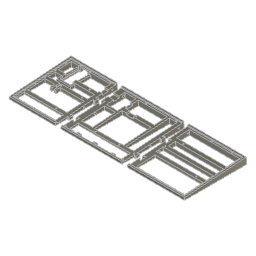
pavilion-x360-keyboard (Autodesk Fusion 360 design; units mm, degrees)
Autodesk Fusion 360 part; units mm, degrees
note: some values were not read from the file. Set by a fixed rule: which face or edge a step refers to.
(part 1 of 2)
ref_plane "WorkPlane3" through (12.125, 0, 0) normal (0, -0.069756, 0.997564) x (1, 0, 0)
sketch "Top" plane through (0, 0, 0) normal (0, -0.069756, 0.997564) x (1, 0, 0)
  line L0 (83, 3) -> (83, 0)
  line L1 (83, 0) -> (0, 0)
  line L2 (0, 0) -> (0, 111.5)
  line L3 (0, 111.5) -> (83, 111.5)
  line L4 (83, 111.5) -> (83, 108.5)
  line L5 (3, 99) -> (4, 99)
  arc A0 (3.9974, 97) -> (4, 99) centre (4, 98) ccw
  line L6 (3.9974, 97) -> (3, 97)
  line L7 (3, 80.5) -> (4, 80.5)
  line L8 (3, 62) -> (4, 62)
  arc A1 (4, 60) -> (4, 62) centre (4, 61) ccw
  line L9 (4, 60) -> (3, 60)
  line L10 (3, 43.5) -> (4, 43.5)
  line L11 (20, 108.5) -> (20, 107.5)
  line L12 (22, 107.5) -> (22, 108.5)
  line L13 (38, 108.5) -> (38, 107.5)
  line L14 (40, 107.5) -> (40, 108.5)
  line L15 (74.5, 108.5) -> (74.5, 107.5)
  line L16 (6.25, 3) -> (6.25, 4)
  line L17 (8.25, 4) -> (8.25, 3)
  line L18 (40.5, 3) -> (40.5, 4)
  line L19 (42.5, 4) -> (42.5, 3)
  line L20 (59.25, 3) -> (59.25, 4)
  line L21 (61.25, 4) -> (61.25, 3)
  line L22 (83, 108.5) -> (76.5, 108.5)
  line L23 (74.5, 108.5) -> (40, 108.5)
  line L24 (38, 108.5) -> (22, 108.5)
  line L25 (20, 108.5) -> (3, 108.5)
  line L26 (3, 108.5) -> (3, 99)
  line L27 (3, 97) -> (3, 80.5)
  line L28 (3, 78.5) -> (3, 62)
  line L29 (3, 60) -> (3, 43.5)
  line L30 (3, 41.5) -> (3, 25)
  line L31 (3, 23) -> (3, 3)
  line L32 (3, 3) -> (6.25, 3)
  line L33 (8.25, 3) -> (21.75, 3)
  line L34 (23.75, 3) -> (40.5, 3)
  line L35 (42.5, 3) -> (59.25, 3)
  line L36 (61.25, 3) -> (83, 3)
  line L37 (93, 3) -> (93, 0)
  line L38 (93, 0) -> (203.25, 0)
  line L39 (203.25, 0) -> (203.25, 3)
  line L40 (97.25, 3) -> (97.25, 4)
  arc A2 (99.25, 4) -> (97.25, 4) centre (98.25, 4) ccw
  line L41 (99.25, 4) -> (99.25, 3)
  line L42 (118.25, 3) -> (118.25, 4)
  arc A3 (120.25, 4) -> (118.25, 4) centre (119.25, 4) ccw
  line L43 (120.25, 4) -> (120.25, 3)
  line L44 (147.75, 3) -> (147.75, 4)
  arc A4 (149.75, 4) -> (147.75, 4) centre (148.75, 4) ccw
  line L45 (149.75, 4) -> (149.75, 3)
  line L46 (181.25, 3) -> (181.25, 4)
  arc A5 (183.25, 4) -> (181.25, 4) centre (182.25, 4) ccw
  line L47 (183.25, 4) -> (183.25, 3)
  line L48 (116.25, 3) -> (116.25, 2.5)
  line L49 (116.25, 2.5) -> (110.25, 2.5)
  line L50 (110.25, 2.5) -> (110.25, 3)
  line L51 (122.25, 3) -> (122.25, 2.5)
  line L52 (122.25, 2.5) -> (145.75, 2.5)
  line L53 (145.75, 2.5) -> (145.75, 3)
  line L54 (179.25, 3) -> (179.25, 2.5)
  line L55 (179.25, 2.5) -> (151.75, 2.5)
  line L56 (151.75, 2.5) -> (151.75, 3)
  line L57 (197.25, 3) -> (197.25, 2.5)
  line L58 (197.25, 2.5) -> (185.25, 2.5)
  line L59 (185.25, 2.5) -> (185.25, 3)
  line L60 (97.25, 3) -> (93, 3)
  line L61 (118.25, 3) -> (116.25, 3)
  line L62 (110.25, 3) -> (99.25, 3)
  line L63 (147.75, 3) -> (145.75, 3)
  line L64 (122.25, 3) -> (120.25, 3)
  line L65 (151.75, 3) -> (149.75, 3)
  line L66 (181.25, 3) -> (179.25, 3)
  line L67 (185.25, 3) -> (183.25, 3)
  line L68 (203.25, 3) -> (201.25, 3)
  line L69 (199.25, 3) -> (197.25, 3)
  line L70 (93, 111.5) -> (203.25, 111.5)
  line L71 (203.25, 111.5) -> (203.25, 108.5)
  line L72 (93, 108.5) -> (93, 111.5)
  line L73 (138.75, 108.5) -> (138.75, 107.5)
  line L74 (140.75, 107.5) -> (140.75, 108.5)
  line L75 (193.25, 108.5) -> (193.25, 107.5)
  line L76 (195.25, 107.5) -> (195.25, 108.5)
  line L77 (138.75, 108.5) -> (93, 108.5)
  line L78 (203.25, 108.5) -> (195.25, 108.5)
  line L79 (193.25, 108.5) -> (140.75, 108.5)
  line L80 (213.25, 108.5) -> (213.25, 111.5)
  line L81 (213.25, 111.5) -> (316.25, 111.5)
  line L82 (316.25, 111.5) -> (316.25, 0)
  line L83 (316.25, 0) -> (213.25, 0)
  line L84 (213.25, 0) -> (213.25, 3)
  line L85 (313.25, 99) -> (312.25, 99)
  line L86 (313.25, 62) -> (312.25, 62)
  line L87 (313.25, 43.5) -> (312.25, 43.5)
  arc A6 (312.25, 43.5) -> (312.2531, 41.5) centre (312.25, 42.5) ccw
  line L88 (312.2531, 41.5) -> (313.25, 41.5)
  line L89 (313.25, 25) -> (312.25, 25)
  arc A7 (312.25, 25) -> (312.25, 23) centre (312.25, 24) ccw
  line L90 (312.25, 23) -> (313.25, 23)
  line L91 (313.25, 99) -> (313.25, 108.5)
  line L92 (313.25, 80.5) -> (313.25, 97)
  line L93 (313.25, 62) -> (313.25, 78.5)
  line L94 (313.25, 3) -> (313.25, 23)
  line L95 (313.25, 25) -> (313.25, 41.5)
  line L96 (313.25, 43.5) -> (313.25, 60)
  line L97 (308, 3) -> (308, 4)
  arc A8 (310, 4) -> (308, 4) centre (309, 4) ccw
  line L98 (310, 4) -> (310, 3)
  line L99 (293.5, 3) -> (293.5, 4)
  arc A9 (295.5, 4) -> (293.5, 4) centre (294.5, 4) ccw
  line L100 (295.5, 4) -> (295.5, 3)
  line L101 (256, 3) -> (256, 4)
  arc A10 (258, 4) -> (256, 4) centre (257, 4) ccw
  line L102 (258, 4) -> (258, 3)
  line L103 (293.5, 108.5) -> (293.5, 107.4999)
  line L104 (295.5, 107.5) -> (295.5, 108.5)
  line L105 (257, 108.5) -> (257, 107.5)
  line L106 (259, 107.5) -> (259, 108.5)
  line L107 (213.25, 3) -> (256, 3)
  line L108 (258, 3) -> (293.5, 3)
  line L109 (295.5, 3) -> (308, 3)
  line L110 (310, 3) -> (313.25, 3)
  line L111 (257, 108.5) -> (213.25, 108.5)
  line L112 (313.25, 108.5) -> (295.5, 108.5)
  line L113 (293.5, 108.5) -> (259, 108.5)
  line L114 (4, 98) -> (312.25, 98) construction
  line L115 (313.25, 111.5) -> (313.25, 0) construction
  arc A11 (312.25, 99) -> (312.2477, 97) centre (312.25, 98) ccw
  line L116 (312.2477, 97) -> (313.25, 97)
  line L117 (4, 79.5) -> (312.25, 79.5) construction
  line L118 (313.25, 80.5) -> (312.25, 80.5)
  line L119 (313.25, 78.5) -> (312.2478, 78.5)
  arc A12 (312.25, 80.5) -> (312.2478, 78.5) centre (312.25, 79.5) ccw
  line L120 (4, 42.5) -> (312.25, 42.5) construction
  line L121 (4, 24) -> (312.25, 24) construction
  line L122 (0, 108.5) -> (316.25, 108.5) construction
  line L123 (0, 3) -> (316.25, 3) construction
  line L124 (3, 0) -> (3, 111.5) construction
  line L125 (93, 2.5) -> (203.25, 2.5) construction
  arc A13 (312.25, 62) -> (312.2508, 60) centre (312.25, 61) ccw
  line L126 (312.2508, 60) -> (313.25, 60)
  line L127 (4, 61) -> (312.25, 61) construction
  arc A14 (20, 107.5) -> (22, 107.5) centre (21, 107.5) ccw
  arc A15 (38, 107.5) -> (40, 107.5) centre (39, 107.5) ccw
  arc A16 (61.25, 4) -> (59.25, 4) centre (60.25, 4) ccw
  arc A17 (293.5, 107.4999) -> (295.5, 107.5) centre (294.5, 107.4999) ccw
  arc A18 (257, 107.5) -> (259, 107.5) centre (258, 107.5) ccw
  line L128 (3, 78.5) -> (4.0035, 78.5)
  arc A19 (4.0035, 78.5) -> (4, 80.5) centre (4, 79.5) ccw
  line L129 (3, 25) -> (4, 25)
  line L130 (3, 23) -> (4.0015, 23)
  line L131 (3, 41.5) -> (3.9975, 41.5)
  arc A20 (3.9975, 41.5) -> (4, 43.5) centre (4, 42.5) ccw
  arc A21 (4.0015, 23) -> (4, 25) centre (4, 24) ccw
  arc A22 (193.25, 107.5) -> (195.25, 107.5) centre (194.25, 107.5) ccw
  arc A23 (138.75, 107.5) -> (140.75, 107.5) centre (139.75, 107.5) ccw
  line L132 (199.25, 3) -> (199.25, 4)
  line L133 (201.25, 3) -> (201.25, 4)
  arc A24 (201.25, 4) -> (199.25, 4) centre (200.25, 4) ccw
  line L134 (76.5, 108.5) -> (76.5, 107.5)
  arc A25 (74.5, 107.5) -> (76.5, 107.5) centre (75.5, 107.5) ccw
  arc A26 (8.25, 4) -> (6.25, 4) centre (7.25, 4) ccw
  arc A27 (42.5, 4) -> (40.5, 4) centre (41.5, 4) ccw
  line L135 (21.75, 3) -> (21.75, 4)
  arc A28 (23.75, 4) -> (21.75, 4) centre (22.75, 4) ccw
  line L136 (23.75, 4) -> (23.75, 3)
  dimension "d87" = 105.5
  dimension "d91" = 3
  dimension "d93" = 1
  dimension "d227" = 1
  dimension "d235" = 1
  dimension "d238" = 1
  dimension "d259" = 1
  dimension "d261" = 1
  dimension "d322" = 1
  dimension "d323" = 1
  dimension "d324" = 1
  dimension "d325" = 4.25
  dimension "d326" = 14.5
  dimension "d327" = 37.5
  dimension "d343" = 10
  dimension "d383" = 2
  dimension "d390" = 2
  dimension "d391" = 2
  dimension "d393" = 100
  dimension "d395" = 3
  dimension "d396" = 1
  dimension "d399" = 1
  dimension "d402" = 1
  dimension "d403" = 2
  dimension "d412" = 3
  dimension "d415" = 3
  dimension "d417" = 0.5
  dimension "d419" = 1
  dimension "d444" = 34.5
  dimension "d445" = 17.75
  dimension "d446" = 9.5
  dimension "d447" = 16.5
  dimension "d448" = 16.5
  dimension "d460" = 1
  dimension "d461" = 1
  dimension "d543" = 1
  dimension "d544" = 17
  dimension "d545" = 2
  dimension "d548" = 16
  dimension "d549" = 2
  dimension "d550" = 34.5
  dimension "d554" = 1
  dimension "d555" = 1
  dimension "d568" = 1
  dimension "d569" = 1
  dimension "d570" = 2
  dimension "d571" = 1
  dimension "d572" = 1
  dimension "d573" = 2
  dimension "d574" = 1
  dimension "d575" = 1
  dimension "d576" = 2
  dimension "d577" = 2
  dimension "d578" = 1
  dimension "d579" = 2
  dimension "d580" = 1
  dimension "d581" = 16.5
  dimension "d582" = 2
  dimension "d583" = 1
  dimension "d585" = 9.5
  dimension "d587" = 1
  dimension "d588" = 2
  dimension "d590" = 1
  dimension "d592" = 16.5
  dimension "d594" = 2
  dimension "d595" = 1
  dimension "d596" = 16.5
  dimension "d598" = 1
  dimension "d600" = 2
  dimension "d601" = 1
  dimension "d602" = 1
  dimension "d603" = 16.5
  dimension "d611" = 1
  dimension "d615" = 2
  dimension "d617" = 1
  dimension "d618" = 2
  dimension "d619" = 16.5
  dimension "d620" = 1
  dimension "d621" = 20
  dimension "d626" = 2
  dimension "d627" = 4.25
  dimension "d628" = 11
  dimension "d629" = 2
  dimension "d630" = 2
  dimension "d631" = 23.5
  dimension "d632" = 2
  dimension "d633" = 2
  dimension "d634" = 27.5
  dimension "d635" = 2
  dimension "d636" = 2
  dimension "d637" = 2
  dimension "d638" = 12
  dimension "d641" = 2
  dimension "d643" = 6
  dimension "d644" = 2
  dimension "d646" = 2
  dimension "d649" = 10
  dimension "d650" = 1
  dimension "d651" = 2
  dimension "d653" = 2
  dimension "d654" = 2
  dimension "d655" = 2
  dimension "d760" = 22.75
  dimension "d762" = 18.75
  dimension "d766" = 1
  dimension "d767" = 4.25
  dimension "d768" = 1
  dimension "d769" = 1
  dimension "d771" = 1
  dimension "d772" = 15.5
  dimension "d773" = 1
  dimension "d774" = 18.75
  dimension "d775" = 1
  dimension "d776" = 9
  dimension "d779" = 2
  dimension "d781" = 46.75
  constraint perpendicular L0 L1
  constraint tangent L5 A0
  constraint coincident L6.end L26
  constraint coincident L7.start L26
  constraint coincident L8.start L26
  constraint tangent L8 A1
  constraint coincident L9.end L26
  constraint coincident L10.start L26
  constraint coincident L1.end L2.start
  constraint coincident L30.start L26
  constraint coincident L30.end L26
  constraint coincident L31.start L26
  constraint coincident L11.start L22
  constraint coincident L12.end L22
  constraint coincident L13.start L22
  constraint coincident L14.end L22
  constraint coincident L15.start L22
  constraint coincident L17.end L32
  constraint coincident L28.start L26
  constraint coincident L33.end L32
  constraint coincident L34.start L32
  constraint coincident L18.start L32
  constraint coincident L19.end L32
  constraint coincident L20.start L32
  constraint coincident L21.end L32
  constraint coincident L40.start L68
  constraint tangent L40 A2
  constraint tangent A2 L41
  constraint coincident L42.start L68
  constraint tangent L42 A3
  constraint tangent A3 L43
  constraint coincident L44.start L68
  constraint tangent L44 A4
  constraint tangent A4 L45
  constraint coincident L46.start L68
  constraint tangent L46 A5
  constraint tangent A5 L47
  constraint coincident L69.start L68
  constraint collinear L1 L38
  constraint coincident L50.end L68
  constraint coincident L53.end L68
  constraint coincident L56.end L68
  constraint coincident L59.end L68
  constraint horizontal L78
  constraint collinear L3 L70
  constraint collinear L37 L72
  constraint collinear L39 L71
  constraint coincident L73.start L78
  constraint coincident L75.start L78
  constraint collinear L77 L78
  constraint collinear L78 L79
  constraint perpendicular L39 L107
  constraint perpendicular L71 L112
  constraint perpendicular L70 L80
  constraint perpendicular L71 L81
  constraint perpendicular L39 L83
  constraint perpendicular L84 L107
  constraint coincident L85.start L94
  constraint coincident L92.start L94
  constraint coincident L86.start L94
  constraint coincident L87.start L94
  constraint tangent L87 A6
  constraint coincident L88.end L94
  constraint coincident L89.start L94
  constraint tangent L89 A7
  constraint tangent A7 L90
  constraint collinear L3 L81
  constraint collinear L1 L83
  constraint collinear L80 L84
  constraint coincident L97.start L107
  constraint vertical L97
  constraint tangent L97 A8
  constraint coincident L98.end L107
  constraint tangent A8 L98
  constraint perpendicular L98 L107
  constraint coincident L99.start L107
  constraint perpendicular L99 L107
  constraint tangent L99 A9
  constraint coincident L100.end L107
  constraint tangent A9 L100
  constraint perpendicular L100 L107
  constraint perpendicular L101 L107
  constraint tangent L101 A10
  constraint coincident L102.end L107
  constraint tangent A10 L102
  constraint perpendicular L102 L107
  constraint coincident L103.start L112
  constraint coincident L105.start L112
  constraint collinear L108 L109
  constraint collinear L109 L110
  constraint collinear L111 L112
  constraint collinear L112 L113
  constraint coincident A0.centre L114.start
  constraint coincident L81 L115.start
  constraint coincident L83 L115.end
  constraint perpendicular L83 L115
  constraint collinear L91 L115
  constraint collinear L92 L115
  constraint collinear L93 L115
  constraint collinear L96 L115
  constraint tangent L85 A11
  constraint coincident L114 A11.centre
  constraint horizontal L117
  constraint tangent L118 A12
  constraint coincident L117 A12.centre
  constraint perpendicular L89 L95
  constraint perpendicular L90 L94
  constraint horizontal L120
  constraint coincident A6.centre L120
  constraint horizontal L114
  constraint horizontal L121
  constraint coincident A7.centre L121
  constraint coincident L3 L124.end
  constraint coincident L2 L122.start
  constraint coincident L2 L123.start
  constraint perpendicular L0 L123
  constraint collinear L32 L123
  constraint coincident L1 L124.start
  constraint perpendicular L3 L124
  constraint collinear L31 L124
  constraint collinear L30 L124
  constraint collinear L29 L124
  constraint perpendicular L2 L122
  constraint collinear L25 L122
  constraint collinear L24 L122
  constraint collinear L0 L4
  constraint collinear L77 L122
  constraint collinear L111 L122
  constraint collinear L60 L123
  constraint collinear L62 L123
  constraint collinear L36 L123
  constraint collinear L61 L123
  constraint collinear L64 L123
  constraint collinear L65 L123
  constraint collinear L66 L123
  constraint collinear L67 L123
  constraint coincident L37 L125.start
  constraint perpendicular L39 L125
  constraint coincident L39 L125.end
  constraint collinear L49 L125
  constraint collinear L52 L125
  constraint collinear L55 L125
  constraint collinear L58 L125
  constraint collinear L69 L123
  constraint collinear L107 L123
  constraint tangent L86 A13
  constraint coincident A1.centre L127
  constraint tangent L11 A14
  constraint tangent L13 A15
  constraint tangent L20 A16
  constraint tangent L103 A17
  constraint tangent L105 A18
  constraint coincident L7.start L124
  constraint tangent L7 A19
  constraint coincident L117.start A19.centre
  constraint coincident A1.centre L127.start
  constraint horizontal L127
  constraint tangent L10 A20
  constraint coincident L120.start A20.centre
  constraint tangent L129 A21
  constraint coincident L121.start A21.centre
  constraint tangent L75 A22
  constraint tangent L76 A22
  constraint tangent L73 A23
  constraint tangent L74 A23
  constraint tangent L14 A15
  constraint tangent L12 A14
  constraint tangent L21 A16
  constraint tangent L132 A24
  constraint tangent L133 A24
  constraint tangent L15 A25
  constraint tangent L134 A25
  constraint tangent L16 A26
  constraint tangent L17 A26
  constraint coincident L82 L122.end
  constraint coincident L114.end A11.centre
  constraint coincident L117.end A12.centre
  constraint coincident A13.centre L127.end
  constraint coincident A6.centre L120.end
  constraint coincident A7.centre L121.end
  constraint coincident L82 L123.end
  constraint tangent L18 A27
  constraint tangent L19 A27
  constraint perpendicular L16 L32
  constraint perpendicular L17 L33
  constraint perpendicular L33 L135
  constraint tangent L135 A28
  constraint perpendicular L18 L34
  constraint perpendicular L19 L35
  constraint perpendicular L20 L35
  constraint perpendicular L21 L36
  constraint tangent A28 L136
  constraint perpendicular L34 L136
  constraint perpendicular L75 L79
  constraint perpendicular L73 L77
  measures "d87" distance of L25.end L31.end
  measures "d91" distance of L4.end L3.end
  measures "d93" distance of L5.start L5.end
  measures "d227" distance of L42.start L42.end
  measures "d235" distance of L44.start L44.end
  measures "d238" distance of L46.start L46.end
  measures "d259" distance of L73.start L73.end
  measures "d261" distance of L75.start L75.end
  measures "d322" distance of L97.start L97.end
  measures "d323" distance of L99.start L99.end
  measures "d324" distance of L101.start L101.end
  measures "d325" distance of L94 A8.centre
  measures "d326" distance of A8.centre A9.centre
  measures "d327" distance of A9.centre A10.centre
  measures "d343" distance of L39 L84
  measures "d383" distance of L101.end A10.start
  measures "d390" distance of L99.end A9.start
  measures "d391" distance of L97.end A8.start
  measures "d393" distance of L83.end L115
  measures "d395" distance of L82 L115
  measures "d396" distance of L85.start L85.end
  measures "d399" distance of L92.start L118.end
  measures "d402" distance of A6.centre L96
  measures "d403" distance of L89.end A7.end
  measures "d412" distance of L2 L124
  measures "d415" vertical distance of L1.end L31.end
  measures "d417" distance of L123 L125.end
  measures "d419" vertical distance of L40.start A2.centre
  measures "d444" distance of L103 L106
  measures "d445" distance of L91 L104
  measures "d446" distance of L85 L122
  measures "d447" distance of L116 L118
  measures "d448" distance of L86 L119
  measures "d460" radius of A7
  measures "d461" distance of A7.centre L115
  measures "d543" distance of L11.start L11.end
  measures "d544" distance of L11 L124
  measures "d545" distance of L11 L12
  measures "d548" distance of L12 L13
  measures "d549" distance of L13 L14
  measures "d550" distance of L14 L15
  measures "d554" distance of L13.start L13.end
  measures "d555" distance of L15.start L15.end
  measures "d568" distance of L18.start L18.end
  measures "d569" distance of L20.start L20.end
  measures "d570" distance of L105 L106
  measures "d571" distance of L106.start L106.end
  measures "d572" distance of L104.start L104.end
  measures "d573" distance of L103 L104
  measures "d574" radius of A18
  measures "d575" radius of A17
  measures "d576" distance of L85 L116
  measures "d577" distance of L118 L119
  measures "d578" distance of L86.start L86.end
  measures "d579" distance of L86 L126
  measures "d580" radius of A13
  measures "d581" distance of L87 L126
  measures "d582" distance of L87 L88
  measures "d583" radius of A6
  measures "d585" distance of L5 L122
  measures "d587" radius of A0
  measures "d588" distance of L5 L6
  measures "d590" distance of L7.start L7.end
  measures "d592" distance of L6 L7
  measures "d594" distance of L7 L128
  measures "d595" radius of A19
  measures "d596" distance of L8 L128
  measures "d598" distance of L8.start L8.end
  measures "d600" distance of L8 L9
  measures "d601" radius of A1
  measures "d602" distance of L10.start L10.end
  measures "d603" distance of L9 L10
  measures "d611" distance of L30.end L129.end
  measures "d615" distance of L129 L130
  measures "d617" radius of A20
  measures "d618" distance of L10 L131
  measures "d619" distance of L129 L131
  measures "d620" radius of A21
  measures "d621" distance of L123 L130
  measures "d626" distance of L75 L76
  measures "d627" distance of L37 L40
  measures "d628" distance of L41 L50
  measures "d629" distance of L42 L48
  measures "d630" distance of L43 L51
  measures "d631" distance of L51 L53
  measures "d632" distance of L44 L53
  measures "d633" distance of L45 L56
  measures "d634" distance of L54 L56
  measures "d635" distance of L46 L54
  measures "d636" distance of L46 L47
  measures "d637" distance of L47 L59
  measures "d638" distance of L57 L59
  measures "d641" distance of L40 L41
  measures "d643" distance of L48 L50
  measures "d644" distance of L44 L45
  measures "d646" distance of L42 L43
  measures "d649" distance of L0 L37
  measures "d650" distance of L69.start L132.end
  measures "d651" distance of L57 L132
  measures "d653" distance of L132 L133
  measures "d654" distance of L39 L133
  measures "d655" distance of L15 L134
  measures "d760" distance of L0 A16.centre
  measures "d762" distance of A16.centre A27.centre
  measures "d766" distance of L16.start L16.end
  measures "d767" distance of L124 A26.centre
  measures "d768" radius of A26
  measures "d769" distance of L33.end L135.end
  measures "d771" radius of A28
  measures "d772" distance of A26.centre A28.centre
  measures "d773" radius of A27
  measures "d774" distance of A27.centre A28.centre
  measures "d775" radius of A16
  measures "d776" distance of L71 A22.centre
  measures "d779" distance of L73 L74
  measures "d781" distance of L72 A23.centre
extrude "Top edges" add sketch "Top" along normal blind 2 makes body 1 at (1, 45.3892, 3.1739) makes body 2 at (147.3333, 0.8313, 0.0581) makes body 3 at (163.1667, 110.2308, 7.7081) makes body 4 at (315.25, 57.0274, 3.9877)
sketch "Middle" plane through (0, 0, 0) normal (0, 0.069756, -0.997564) x (-1, 0, 0)
  line L0 (-83, 0) -> (0, 0)
  line L1 (0, 0) -> (0, 111.5)
  line L2 (0, 111.5) -> (-83, 111.5)
  line L3 (-77, 6) -> (-6, 6)
  line L4 (-6, 105.5) -> (-77, 105.5)
  line L5 (-83, 0) -> (0, 0)
  line L6 (0, 111.5) -> (-83, 111.5)
  line L7 (-6, 82.5) -> (-77, 82.5)
  line L8 (-77, 76.5) -> (-6, 76.5)
  line L9 (-6, 21) -> (-77, 21)
  line L10 (-77, 27) -> (-6, 27)
  line L11 (-77, 64) -> (-6, 64)
  line L12 (-6, 6) -> (-6, 21)
  line L13 (-6, 27) -> (-6, 58)
  line L14 (-6, 64) -> (-6, 76.5)
  line L15 (-6, 82.5) -> (-6, 105.5)
  line L16 (-83, 111.5) -> (-83, 0)
  line L17 (-77, 21) -> (-77, 6)
  line L18 (-77, 58) -> (-77, 27)
  line L19 (-77, 105.5) -> (-77, 82.5)
  line L20 (-77, 76.5) -> (-77, 64)
  circle A0 centre (-65.25, 79.5) radius 1
  circle A1 centre (-32.25, 61) radius 1
  circle A2 centre (-69.75, 61) radius 1
  circle A3 centre (-60.25, 24) radius 1
  line L21 (-93, 111.5) -> (-93, 0)
  line L22 (-203.25, 111.5) -> (-93, 111.5)
  line L23 (-203.25, 111.5) -> (-203.25, 0)
  line L24 (-203.25, 0) -> (-93, 0) construction
  line L25 (-213.25, 111.5) -> (-213.25, 0)
  line L26 (-316.25, 111.5) -> (-213.25, 111.5)
  line L27 (-213.25, 0) -> (-316.25, 0)
  line L28 (-219.25, 105.5) -> (-310.25, 105.5)
  line L29 (-310.25, 6) -> (-223.25, 6)
  line L30 (-219.25, 82.5) -> (-310.25, 82.5)
  line L31 (-223.25, 76.5) -> (-310.25, 76.5)
  line L32 (-223.25, 64) -> (-310.25, 64)
  line L33 (-219.25, 58) -> (-310.25, 58)
  line L34 (-219.25, 82.5) -> (-219.25, 105.5)
  line L35 (-219.25, 64) -> (-219.25, 76.5) construction
  line L36 (-310.25, 39.5) -> (-310.25, 6)
  line L37 (-310.25, 105.5) -> (-310.25, 82.5)
  line L38 (-310.25, 76.5) -> (-310.25, 64)
  circle A4 centre (-234.75, 79.5) radius 1
  circle A5 centre (-201, 24) radius 1
  line L39 (-103, 21) -> (-197.25, 21)
  line L40 (-197.25, 105.5) -> (-197.25, 27)
  line L41 (-122.25, 2.5) -> (-122.25, 7.5)
  line L42 (-145.75, 2.5) -> (-145.75, 7.5)
  line L43 (-179.25, 2.5) -> (-179.25, 6.5)
  line L44 (-197.25, 2.5) -> (-197.25, 21)
  line L45 (-110.25, 6) -> (-103, 6)
  line L46 (-110.25, 2.5) -> (-116.25, 2.5)
  line L47 (-122.25, 2.5) -> (-145.75, 2.5)
  line L48 (-110.25, 2.5) -> (-110.25, 6)
  line L49 (-151.75, 2.5) -> (-151.75, 7.5)
  line L50 (-185.25, 2.5) -> (-185.25, 6.5)
  line L51 (-116.25, 2.5) -> (-116.25, 7.5)
  line L52 (-116.25, 7.5) -> (-122.25, 7.5)
  line L53 (-145.75, 7.5) -> (-151.75, 7.5)
  line L54 (-179.25, 6.5) -> (-185.25, 6.5)
  line L55 (-183.25, 105.5) -> (-183.25, 27)
  line L56 (-197.25, 105.5) -> (-183.25, 105.5)
  line L57 (-183.25, 27) -> (-197.25, 27)
  line L58 (-179.25, 105.5) -> (-127, 105.5)
  line L59 (-123, 105.5) -> (-103, 105.5)
  line L60 (-103, 27) -> (-123, 27)
  line L61 (-127, 27) -> (-179.25, 27)
  line L62 (-103, 72.25) -> (-123, 72.25)
  line L63 (-103, 68.25) -> (-123, 68.25)
  line L64 (-123, 105.5) -> (-123, 72.25)
  line L65 (-123, 68.25) -> (-123, 27)
  line L66 (-316.25, 0) -> (-316.25, 111.5)
  circle A6 centre (-220.5, 61) radius 1
  line L67 (-316.25, 111.5) -> (-316.25, 0)
  line L68 (-313.25, 111.5) -> (-313.25, 0) construction
  line L69 (-219.25, 45.5) -> (-310.25, 45.5)
  line L70 (-223.25, 39.5) -> (-310.25, 39.5)
  line L71 (-219.25, 45.5) -> (-219.25, 58)
  line L72 (-310.25, 58) -> (-310.25, 45.5)
  circle A7 centre (-294.5, 42.5) radius 1
  line L73 (-219.25, 111.5) -> (-219.25, 0) construction
  line L74 (0, 111.5) -> (0, 0) construction
  line L75 (-223.25, 76.5) -> (-223.25, 64)
  line L76 (-219.25, 76.5) -> (-223.25, 76.5) construction
  line L77 (-219.25, 64) -> (-223.25, 64) construction
  line L78 (-223.25, 39.5) -> (-223.25, 6)
  line L79 (-103, 72.25) -> (-103, 105.5)
  line L80 (-103, 68.25) -> (-103, 27)
  line L81 (-103, 21) -> (-103, 6)
  line L82 (-3, 0) -> (-3, 111.5) construction
  line L83 (0, 0) -> (0, 111.5)
  line L84 (-4, 61) -> (-312.25, 61) construction
  line L85 (-4, 79.5) -> (-312.25, 79.5) construction
  line L86 (-4, 24) -> (-312.25, 24) construction
  line L87 (-93, 111.5) -> (-203.25, 111.5)
  line L88 (-93, 2.5) -> (-203.25, 2.5) construction
  line L89 (-93, 0) -> (-203.25, 0)
  line L90 (-4, 42.5) -> (-312.25, 42.5) construction
  line L91 (-151.75, 2.5) -> (-179.25, 2.5)
  line L92 (-185.25, 2.5) -> (-197.25, 2.5)
  line L93 (-23.5, 58) -> (-23.5, 50)
  line L94 (-23.5, 50) -> (-33.5, 50)
  line L95 (-33.5, 50) -> (-33.5, 58)
  line L96 (-6, 58) -> (-23.5, 58)
  line L97 (-33.5, 58) -> (-77, 58)
  line L98 (-127, 82.5) -> (-179.25, 82.5)
  line L99 (-127, 76.5) -> (-179.25, 76.5)
  line L100 (-127, 105.5) -> (-127, 82.5)
  line L101 (-127, 76.5) -> (-127, 27)
  line L102 (-179.25, 105.5) -> (-179.25, 82.5)
  line L103 (-179.25, 76.5) -> (-179.25, 27)
  circle A8 centre (-149.75, 79.5) radius 1
  circle A9 centre (-65.25, 79.5) radius 1.75
  circle A10 centre (-149.75, 79.5) radius 1.75
  circle A11 centre (-234.75, 79.5) radius 1.75
  circle A12 centre (-32.25, 61) radius 1.75
  circle A13 centre (-69.75, 61) radius 1.75
  circle A14 centre (-220.5, 61) radius 1.75
  circle A15 centre (-60.25, 24) radius 1.75
  circle A16 centre (-201, 24) radius 1.75
  circle A17 centre (-294.5, 42.5) radius 1.75
  point P0 (-93, 0)
  point P1 (-93, 111.5)
  point P2 (-203.25, 111.5)
  point P3 (-203.25, 0)
  point P4 (-213.25, 0)
  point P5 (-116.25, 2.5)
  point P6 (-110.25, 2.5)
  point P7 (-122.25, 2.5)
  point P8 (-145.75, 2.5)
  point P9 (-151.75, 2.5)
  point P10 (-197.25, 2.5)
  point P11 (-185.25, 2.5)
  dimension "d142" = 6
  dimension "d152" = 6
  dimension "d153" = 6
  dimension "d154" = 6
  dimension "d159" = 6
  dimension "d160" = 6
  dimension "d163" = 2
  dimension "d164" = 2
  dimension "d166" = 2
  dimension "d168" = 2
  dimension "d332" = 6
  dimension "d346" = 2
  dimension "d350" = 2
  dimension "d351" = 3.75
  dimension "d359" = 14
  dimension "d360" = 4
  dimension "d361" = 4
  dimension "d363" = 4
  dimension "d379" = 6
  dimension "d385" = 2
  dimension "d404" = 78.5
  dimension "d405" = 92.75
  dimension "d406" = 6
  dimension "d407" = 2
  dimension "d408" = 18.75
  dimension "d409" = 6
  dimension "d506" = 4
  dimension "d507" = 4
  dimension "d511" = 10
  dimension "d512" = 10
  dimension "d515" = 10
  dimension "d657" = 57.25
  dimension "d658" = 6
  dimension "d659" = 23
  dimension "d660" = 12.5
  dimension "d662" = 29.25
  dimension "d663" = 66.75
  dimension "d664" = 62.25
  dimension "d665" = 31
  dimension "d666" = 15
  dimension "d667" = 6
  dimension "d668" = 6
  dimension "d669" = 33.25
  dimension "d673" = 41.25
  dimension "d674" = 20
  dimension "d679" = 7.25
  dimension "d680" = 6
  dimension "d681" = 23.5
  dimension "d682" = 6
  dimension "d683" = 6
  dimension "d684" = 27.5
  dimension "d685" = 6
  dimension "d686" = 12.5
  dimension "d705" = 6
  dimension "d708" = 6
  dimension "d710" = 7.5
  dimension "d730" = 52.25
  dimension "d802" = 8
  dimension "d803" = 17.5
  dimension "d804" = 10
  dimension "d814" = 2
  dimension "d817" = 56.75
  dimension "d827" = 6.5
  dimension "d830" = 3.5
  dimension "d831" = 3.5
  dimension "d832" = 3.5
  dimension "d833" = 3.5
  dimension "d834" = 3.5
  dimension "d835" = 3.5
  dimension "d836" = 3.5
  dimension "d837" = 3.5
  dimension "d844" = 3.5
  constraint coincident L0.start L5.start
  constraint perpendicular L3 L12
  constraint coincident L2.end L6.end
  constraint coincident L0.end L1.start
  constraint coincident L1.end L2.start
  constraint coincident L7.start L12
  constraint coincident L8.end L12
  constraint perpendicular L9 L12
  constraint coincident L10.end L12
  constraint perpendicular L10 L12
  constraint coincident L13.end L12
  constraint perpendicular L12 L96
  constraint coincident L11.end L12
  constraint perpendicular L11 L12
  constraint collinear L12 L13
  constraint collinear L13 L14
  constraint collinear L14 L15
  constraint collinear L17 L19
  constraint collinear L18 L19
  constraint collinear L19 L20
  constraint coincident P1 L21.start
  constraint coincident P0 L21.end
  constraint coincident P2 L22.start
  constraint coincident P3 L23.end
  constraint perpendicular L30 L37
  constraint coincident L31.end L37
  constraint coincident L33.end L37
  constraint collinear L7 L30
  constraint collinear L8 L31
  constraint collinear L11 L32
  constraint collinear L33 L96
  constraint collinear L36 L37
  constraint collinear L37 L72
  constraint collinear L37 L38
  constraint collinear L6 L26
  constraint collinear L5 L27
  constraint coincident L25 P4
  constraint coincident L39.end L40
  constraint collinear L9 L39
  constraint coincident P5 L46.end
  constraint coincident P6 L46.start
  constraint coincident P7 L41.start
  constraint coincident P8 L42.start
  constraint coincident P9 L49.start
  constraint coincident P11 L50.start
  constraint coincident P10 L44.start
  constraint coincident L55.end L60
  constraint coincident L58.start L56
  constraint coincident L59.start L58
  constraint coincident L61.start L60
  constraint coincident L63.end L64
  constraint collinear L100 L101
  constraint perpendicular L26 L66
  constraint collinear L66 L67
  constraint perpendicular L69 L72
  constraint coincident L36.start L72
  constraint collinear L36 L72
  constraint coincident L26 L73.start
  constraint coincident L27 L73.end
  constraint perpendicular L27 L73
  constraint collinear L71 L73
  constraint collinear L35 L73
  constraint collinear L34 L73
  constraint perpendicular L32 L75
  constraint collinear L8 L76
  constraint collinear L11 L77
  constraint perpendicular L29 L78
  constraint coincident A1.centre L84
  constraint coincident A2.centre L84
  constraint coincident A0.centre L85
  constraint coincident A3.centre L86
  constraint collinear L64 L65
  constraint collinear L60 L61
  constraint collinear L57 L61
  constraint coincident A5.centre L86
  constraint coincident A6.centre L84
  constraint coincident A4.centre L85
  constraint perpendicular L51 L52
  constraint collinear L52 L53
  constraint coincident L43.start L88
  constraint coincident A7.centre L90
  constraint perpendicular L43 L91
  constraint coincident L95.end L96
  constraint collinear L96 L97
  constraint perpendicular L93 L94
  constraint perpendicular L98 L102
  constraint coincident L99.start L100
  constraint perpendicular L99 L102
  constraint collinear L7 L98
  constraint collinear L8 L99
  constraint collinear L102 L103
  constraint coincident L85 A8.centre
  constraint concentric A0 A9
  constraint concentric A8 A10
  constraint concentric A4 A11
  constraint concentric A1 A12
  constraint concentric A2 A13
  constraint concentric A6 A14
  constraint concentric A3 A15
  constraint concentric A5 A16
  constraint concentric A7 A17
  measures "d142" distance of L1 L12
  measures "d152" distance of L7.end L8.start
  measures "d153" distance of L9.end L10.start
  measures "d154" distance of L18.start L11.start
  measures "d159" distance of L16 L19
  measures "d160" distance of L3 L5
  measures "d163" diameter of A0
  measures "d164" diameter of A1
  measures "d166" diameter of A2
  measures "d168" diameter of A3
  measures "d332" distance of L27 L29
  measures "d346" diameter of A4
  measures "d350" diameter of A5
  measures "d351" distance of A5.centre L40
  measures "d359" distance of L40 L55
  measures "d360" distance of L55 L102
  measures "d361" distance of L64 L100
  measures "d363" distance of L62 L63
  measures "d379" distance of L37 L66
  measures "d385" diameter of A6
  measures "d404" distance of A4.centre L68
  measures "d405" distance of A6.centre L68
  measures "d406" distance of L69 L70
  measures "d407" diameter of A7
  measures "d408" distance of L68 A7.centre
  measures "d409" distance of L25 L73
  measures "d506" horizontal distance of L30.start L31.start
  measures "d507" horizontal distance of L69.start L70.start
  measures "d511" distance of L21 L79
  measures "d512" distance of L21 L80
  measures "d515" distance of L21 L81
  measures "d657" distance of A3.centre L82
  measures "d658" distance of L4 L6
  measures "d659" distance of L4 L7
  measures "d660" distance of L8 L11
  measures "d662" distance of A1.centre L82
  measures "d663" distance of A2.centre L82
  measures "d664" distance of A0.centre L82
  measures "d665" distance of L10 L96
  measures "d666" distance of L3 L9
  measures "d667" distance of L59 L87
  measures "d668" distance of L56 L87
  measures "d669" distance of L59 L62
  measures "d673" distance of L60 L63
  measures "d674" distance of L64 L79
  measures "d679" distance of L48 L81
  measures "d680" distance of L48 L51
  measures "d681" distance of L41 L42
  measures "d682" distance of L41 L51
  measures "d683" distance of L42 L49
  measures "d684" distance of L43 L49
  measures "d685" distance of L26 L28
  measures "d686" distance of L33 L69
  measures "d705" distance of L43 L50
  measures "d708" distance of L24 L45
  measures "d710" distance of L52 L89
  measures "d730" distance of L100 L102
  measures "d802" distance of L95.end L94.end
  measures "d803" distance of L13 L93
  measures "d804" distance of L93 L95
  measures "d814" diameter of A8
  measures "d817" distance of L21 A8.centre
  measures "d827" distance of L24 L54
  measures "d830" diameter of A9
  measures "d831" diameter of A10
  measures "d832" diameter of A11
  measures "d833" diameter of A12
  measures "d834" diameter of A13
  measures "d835" diameter of A14
  measures "d836" diameter of A15
  measures "d837" diameter of A16
  measures "d844" diameter of A17
extrude "Main body" add sketch "Middle" along normal blind 2 contours L0 L1 L2 L5 L6 L16 L83 | L21 L22 L23 L87 L89 | L25 L26 L27 L66 L67 | A9 | A10 | A11 | A12 | A13 | A14 | A15 | A16 | A17 bodies 2 1 4 3
draft "Front draft" angle 8 neutral plane through (0, -0.1395, 1.9951) pull (0, -0.069756, 0.997564) 4 faces at (55.3333, 0.093, -1.3301) (166.5, 0, 0) (281.9167, 0.0465, -0.665) (247.5833, -0.093, 1.3301) on bodies 1 2 4
draft "Bottom draft" angle 4 neutral plane through (41.5, -0.2804, -0.0196) pull (0, -0.997564, 0.069756) 3 faces at (219.9167, 15.0823, -0.9502) (96.3333, 59.7233, 2.1714) (29.6667, 1.7608, -1.8818) on bodies 1 2 4
sketch "Slots" plane through (0, 0, 0) normal (0, -0.069756, 0.997564) x (1, 0, 0)
  line L0 (197.25, 105.5) -> (197.25, 27)
  line L1 (197.25, 27) -> (183.25, 27)
  line L2 (183.25, 27) -> (183.25, 105.5)
  line L3 (183.25, 105.5) -> (197.25, 105.5)
  circle A0 centre (201, 24) radius 1
  line L4 (123, 68.25) -> (123, 27)
  line L5 (123, 27) -> (103, 27)
  line L6 (103, 27) -> (103, 68.25)
  line L7 (103, 68.25) -> (123, 68.25)
  line L8 (123, 105.5) -> (123, 72.25)
  line L9 (123, 72.25) -> (103, 72.25)
  line L10 (103, 72.25) -> (103, 105.5)
  line L11 (103, 105.5) -> (123, 105.5)
  line L12 (132, 27) -> (174.25, 27)
  line L13 (174.25, 27) -> (174.25, 21)
  line L14 (174.25, 21) -> (132, 21)
  line L15 (132, 21) -> (132, 27)
  line L16 (77, 82.5) -> (77, 105.5) construction
  line L17 (77, 95) -> (127, 95)
  line L18 (127, 95) -> (127, 85)
  line L19 (127, 85) -> (77, 85)
  line L20 (77, 85) -> (77, 95)
  line L21 (6, 64) -> (77, 64) construction
  line L22 (27, 64) -> (30, 64)
  line L23 (30, 64) -> (30, 58)
  line L24 (30, 58) -> (27, 58)
  line L25 (27, 58) -> (27, 64)
  line L26 (26.5, 58) -> (30.5, 58)
  line L27 (30.5, 58) -> (30.5, 50)
  line L28 (30.5, 50) -> (26.5, 50)
  line L29 (26.5, 50) -> (26.5, 58)
  line L30 (33.5, 50) -> (23.5, 50)
  line L31 (23.5, 50) -> (23.5, 58) construction
  line L32 (127, 105.5) -> (127, 82.5) construction
  line L33 (6, 58) -> (23.5, 58) construction
  line L34 (127, 27) -> (179.25, 27) construction
  line L35 (103, 21) -> (197.25, 21) construction
  line L36 (127, 82.5) -> (179.25, 82.5) construction
  line L37 (127, 76.5) -> (179.25, 76.5) construction
  circle A1 centre (149.75, 79.5) radius 1 construction
  line L38 (134.5, 82.5) -> (147, 82.5)
  line L39 (147, 82.5) -> (147, 76.5)
  line L40 (147, 76.5) -> (134.5, 76.5)
  line L41 (134.5, 76.5) -> (134.5, 82.5)
  dimension "d789" = 10
  dimension "d791" = 10.5
  dimension "d800" = 3
  dimension "d805" = 4
  dimension "d806" = 3
  dimension "d807" = 3.5
  dimension "d828" = 20
  dimension "d829" = 12.5
  constraint perpendicular L12 L15
  constraint perpendicular L13 L14
  constraint coincident L16 L17.start
  constraint collinear L16 L20
  constraint perpendicular L17 L20
  constraint perpendicular L19 L20
  constraint coincident L21 L22.start
  constraint coincident L21 L22.end
  constraint perpendicular L22 L25
  constraint collinear L28 L30
  constraint collinear L18 L32
  constraint collinear L26 L33
  constraint collinear L24 L33
  constraint collinear L12 L34
  constraint collinear L14 L35
  constraint coincident L37 L39.end
  constraint coincident L36 L38.start
  constraint collinear L36 L38
  constraint collinear L37 L40
  measures "d789" distance of L17.end L18.end
  measures "d791" distance of L16.end L17
  measures "d800" distance of L23 L25
  measures "d805" distance of L27 L29
  measures "d806" distance of L29 L31
  measures "d807" distance of L25 L31
  measures "d828" distance of L32 L39
  measures "d829" distance of L39 L41
extrude "FCP slots" cut sketch "Slots" against normal blind 0.75 contours L12 L13 L14 L15 bodies 2
extrude "Wire slot" cut sketch "Slots" against normal blind 3 contours L8 L17 L18 L19 | L10 L17 L19 L20 | L22 L23 L24 L25 L26 | L38 L39 L40 L41 bodies 2 1
extrude "Threaded inserts - 1" cut sketch "Middle" along normal through all from surface at 3.5 contours A9 | A10 | A11 bodies 2 1 4
extrude "Threaded inserts - 2" cut sketch "Middle" along normal through all from surface at 4.3 contours A12 | A13 | A14 bodies 1 4
extrude "Threaded inserts - 3" cut sketch "Middle" along normal through all from surface at 3 contours A17 bodies 4
extrude "Threaded inserts - 4" cut sketch "Middle" along normal through all from surface at 1.7 contours A15 | A16 bodies 2 1
extrude "LED slot" cut sketch "Slots" against normal through all contours L24 L26 L27 L28 L29 L30 bodies 1
sketch "Bottom" plane through (0, 0, -2.0343) normal (0, 0, -1) x (1, 0, 0)
  line L0 (77, -82.8437) -> (77, -105.8999)
  line L1 (77, -105.8999) -> (6, -105.8999)
  line L2 (83, 0.4213) -> (0, 0.4213)
  line L3 (0, -111.9145) -> (83, -111.9145) construction
  line L4 (38, -105.8999) -> (38, -71.8999)
  line L5 (38, -71.8999) -> (19, -71.8999)
  line L6 (19, -71.8999) -> (19, -105.8999)
  line L7 (41, -105.8999) -> (41, -68.8999)
  line L8 (41, -68.8999) -> (16, -68.8999)
  line L9 (16, -68.8999) -> (16, -105.8999)
  line L10 (83, -72.5638) -> (87, -74.8732)
  line L11 (87, -74.8732) -> (87, -66.2544)
  line L12 (87, -66.2544) -> (83, -68.5638)
  line L13 (83, -111.9145) -> (83, 0.4213) construction
  line L14 (0, -70.5638) -> (316.25, -70.5638) construction
  line L15 (93, 0.4213) -> (93, -111.9145)
  line L16 (77, -21.1935) -> (6, -21.1935) construction
  line L17 (0, -24.2009) -> (316.25, -24.2009) construction
  line L18 (83, -26.2009) -> (87, -28.5103)
  line L19 (87, -28.5103) -> (87, -19.8915)
  line L20 (87, -19.8915) -> (83, -22.2009)
  line L21 (93, -73.1888) -> (97.25, -75.6425)
  line L22 (93, -67.9388) -> (97.25, -65.4851)
  line L23 (97.25, -65.4851) -> (97.25, -75.6425)
  line L24 (93, -26.8259) -> (97.25, -29.2796)
  line L25 (97.25, -29.2796) -> (97.25, -19.1221)
  line L26 (97.25, -19.1221) -> (93, -21.5759)
  line L27 (213.25, -73.1888) -> (217.5, -75.6425)
  line L28 (217.5, -65.4851) -> (217.5, -75.6425)
  line L29 (213.25, -67.9388) -> (217.5, -65.4851)
  line L30 (213.25, -21.5759) -> (217.5, -19.1221)
  line L31 (217.5, -19.1221) -> (217.5, -29.2796)
  line L32 (213.25, -26.8259) -> (217.5, -29.2796)
  line L33 (203.25, -111.9145) -> (203.25, 0.4213) construction
  line L34 (203.25, -72.5638) -> (207.25, -74.8732)
  line L35 (207.25, -66.2544) -> (203.25, -68.5638)
  line L36 (203.25, -26.2009) -> (207.25, -28.5103)
  line L37 (207.25, -28.5103) -> (207.25, -19.8915)
  line L38 (207.25, -19.8915) -> (203.25, -22.2009)
  line L39 (77, -105.8999) -> (6, -105.8999)
  line L40 (20, -72.8999) -> (37, -72.8999)
  line L41 (37, -72.8999) -> (37, -105.8999)
  line L42 (28.5, -68.8999) -> (28.5, -111.9145) construction
  line L43 (21.75, -111.9145) -> (35.25, -111.9145)
  line L44 (35.25, -111.9145) -> (35.25, -105.8999)
  line L45 (21.75, -105.8999) -> (21.75, -111.9145)
  line L46 (83, -111.9145) -> (0, -111.9145)
  line L47 (77, -76.8291) -> (6, -76.8291) construction
  line L48 (20, -72.8999) -> (20, -105.8999)
  line L49 (38, -105.8999) -> (19, -105.8999)
  line L50 (83, -72.5638) -> (83, -68.5638)
  line L51 (83, -26.2009) -> (83, -22.2009)
  line L52 (213.25, 0.4213) -> (213.25, -111.9145) construction
  line L53 (203.25, -72.5638) -> (203.25, -68.5638)
  line L54 (203.25, -22.2009) -> (203.25, -26.2009)
  line L55 (93, -26.8259) -> (93, -21.5759)
  line L56 (93, -73.1888) -> (93, -67.9388)
  line L57 (213.25, -73.1888) -> (213.25, -67.9388)
  line L58 (213.25, -26.8259) -> (213.25, -21.5759)
  line L59 (0, 0.4213) -> (0, -111.9145) construction
  line L60 (316.25, -111.9145) -> (316.25, 0.4213)
  line L61 (213.25, -72.5638) -> (217.25, -74.8732) construction
  line L62 (217.25, -74.8732) -> (217.25, -66.2544) construction
  line L63 (217.25, -66.2544) -> (213.25, -68.5638) construction
  line L64 (207.25, -74.8732) -> (207.25, -66.2544)
  line L65 (6, -27.2082) -> (77, -27.2082) construction
  ellipse E0 centre (65.25, -79.8364) end of major axis (65.25, -81.5907) minor radius 1.75
  ellipse E1 centre (69.75, -61.2912) end of major axis (69.75, -63.0455) minor radius 1.75
  ellipse E2 centre (32.25, -61.2912) end of major axis (32.25, -63.0455) minor radius 1.75
  ellipse E3 centre (60.25, -24.2009) end of major axis (60.25, -25.9551) minor radius 1.75
  dimension "d170" = 19
  dimension "d177" = 36
  dimension "d271" = 4
  dimension "d286" = 4
  dimension "d287" = 60
  dimension "d477" = 60
  dimension "d481" = 5.25
  dimension "d509" = 60
  dimension "d518" = 4
  dimension "d522" = 4
  dimension "d523" = 4
  dimension "d524" = 25
  dimension "d526" = 37
  dimension "d527" = 3
  dimension "d529" = 1
  dimension "d530" = 1
  dimension "d533" = 13.5
  dimension "d538" = 4
  dimension "d539" = 60
  dimension "d690" = 6.2653
  dimension "d691" = 1
  dimension "d694" = 4
  dimension "d695" = 60
  dimension "d699" = 60
  dimension "d700" = 4.25
  dimension "d701" = 60
  dimension "d735" = 4
  dimension "d736" = 4
  dimension "d737" = 0.25
  dimension "d738" = 0.5413
  dimension "d825" = 4
  dimension "d826" = 60
  constraint coincident L1 L6.end
  constraint coincident L13 L18.start
  constraint coincident L13 L20.end
  constraint coincident L15 L21.start
  constraint coincident L15 L22.start
  constraint coincident L15 L24.start
  constraint coincident L15 L26.end
  constraint symmetric L14 L21 L22
  constraint symmetric L14 L27 L29
  constraint symmetric L17 L30 L32
  constraint symmetric L17 L24 L26
  constraint coincident L33 L34.start
  constraint coincident L33 L35.end
  constraint coincident L33 L36.start
  constraint coincident L33 L38.end
  constraint symmetric L17 L36 L38
  constraint perpendicular L4 L40
  constraint coincident L39 L41.end
  constraint perpendicular L39 L41
  constraint midpoint L8 L42.start
  constraint coincident L3 L42.end
  constraint perpendicular L3 L42
  constraint collinear L3 L43
  constraint midpoint L42.end L43
  constraint perpendicular L43 L45
  constraint symmetric L17 L18 L20
  constraint symmetric L10 L12 L14
  constraint coincident L10.start L13
  constraint coincident L12.end L13
  constraint coincident L4.start L39
  constraint coincident L1 L9.end
  constraint coincident L7.start L39
  constraint coincident L39 L48.end
  constraint coincident L39 L44.end
  constraint coincident L39 L45.start
  constraint coincident L29.start L52
  constraint coincident L27.start L52
  constraint coincident L32.start L52
  constraint coincident L30.start L52
  constraint coincident L14.start L59
  constraint coincident L17.start L59
  constraint coincident L14.end L60
  constraint coincident L17.end L60
  constraint coincident L57 L63.end
  constraint coincident L61.end L62.start
  constraint coincident L62.end L63.start
  constraint equal L34 L61
  constraint equal L35 L63
  constraint vertical L62
  constraint equal L28 L31
  constraint equal L27 L32
  constraint vertical L31
  constraint symmetric L14 L61 L63
  constraint equal L21 L27
  constraint equal L23 L28
  constraint vertical L23
  constraint symmetric L14 L34 L35
  constraint vertical L25
  constraint equal L23 L25
  constraint equal L21 L24
  constraint symmetric L16 L17 L65
  measures "d170" distance of L6.end L4.start
  measures "d177" distance of L0 L7
  measures "d271" distance of L10.start L12.end
  measures "d286" distance of L18.start L20.end
  measures "d287" angle of L13 L18
  measures "d477" angle of L15 L21
  measures "d481" distance of L27.start L29.start
  measures "d509" angle of L15 L24
  measures "d518" distance of L34.start L35.end
  measures "d522" distance of L36.start L38.end
  measures "d523" distance of L33 L37
  measures "d524" distance of L7 L9
  measures "d526" distance of L1 L8
  measures "d527" distance of L5 L8
  measures "d529" distance of L4 L41
  measures "d530" distance of L5 L40
  measures "d533" distance of L44 L45
  measures "d538" distance of L13 L19
  measures "d539" angle of L10 L13
  measures "d690" distance of L14 L47
  measures "d691" distance of L6 L48
  measures "d694" distance of L11 L50
  measures "d695" angle of L27 L28
  measures "d699" angle of L31 L32
  measures "d700" distance of L28 L52
  measures "d701" angle of L36 L37
  measures "d735" distance of L63.end L61.start
  measures "d736" distance of L52 L62
  measures "d737" distance of L28 L62
  measures "d738" distance of L27 L61
  measures "d825" distance of L53 L64
  measures "d826" angle of L34 L64
extrude "Chip bracket" add sketch "Bottom" against normal blind 5 contours L1 L4 L5 L6 L7 L8 L9 L39 bodies 1
extrude "Chip hole" cut sketch "Bottom" against normal through all contours L1 L4 L5 L6 L39 L40 L41 L48 L49 | L1 L39 L40 L41 L48 L49 bodies 1
extrude "Chip base" add sketch "Bottom" against normal blind 2.5 contours L1 L4 L5 L6 L39 L40 L41 L48 L49 bodies 1
extrude "Port hole" cut sketch "Bottom" against normal blind 7.5 contours L1 L39 L43 L44 L45 L46 L49 bodies 1
extrude "Joints - female" cut sketch "Bottom" along normal up to surface contours L15 L24 L25 L26 L55 | L15 L21 L22 L23 L56 | L27 L28 L29 L57 | L30 L31 L32 L58 end surface through (0, 0, 0) normal (0, -0.069756, 0.997564) offset 0 bodies 2 4
extrude "Joints - male" add sketch "Bottom" along normal up to surface contours L10 L11 L12 L50 | L18 L19 L20 L51 | L34 L35 L53 L64 | L36 L37 L38 L54 end surface through (0, 0, 0) normal (0, -0.069756, 0.997564) offset 0 bodies 2 1